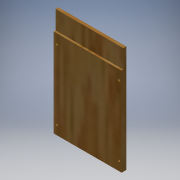
# Autodesk Inventor part: arduinoShelf
Saved by Autodesk Inventor 2016 (Build 200138000, 138)
## iProperties
Created: 2015-10-11
Part Number: arduinoShelf
Material: Plywood, Sheathing
Document SubType Name: Modeling
Designer: Artur
Density: 0.552 g/cm^3
Appearance: Plywood - New
Mass: 22.4443 g
Surface Area: 193.1 cm^2
Volume: 40.66 cm^3
Author: Artur
Autodesk Inventor part; units mm, degrees
ref_plane "YZ Plane" through (0, 0, 0) normal (1, 0, 0) x (0, 1, 0)
ref_plane "XZ Plane" through (0, 0, 0) normal (0, 1, 0) x (-1, 0, 0)
ref_plane "XY Plane" through (0, 0, 0) normal (0, 0, 1) x (1, 0, 0)
sketch "Sketch1" plane through (0, 0, 0) normal (0, 1, 0) x (-1, 0, 0)
  line L0 (0, 0) -> (-73, 0)
  line L1 (-73, 0) -> (-73, -115)
  line L2 (-73, -115) -> (0, -115)
  line L3 (0, -115) -> (0, 0)
  dimension "d0" = 115
  dimension "d1" = 73
  constraints: 8 end point, 2 parallel, 1 horizontal, 1 perpendicular
  measures "d0" distance of L2.end L0.start
  measures "d1" distance of L0.start L0.end
extrude "Extrusion1" add sketch "Sketch1" along normal blind 5
sketch "Sketch2" plane through (73, 0, 0) normal (1, 0, 0) x (0, 0, -1)
  line L0 (0, 0) -> (0, 5) construction
  line L1 (0, 0) -> (115, 0) construction
  line L2 (0, 2) -> (20, 2)
  line L3 (20, 2) -> (20, 0)
  line L4 (0, 2) -> (0, 0)
  line L5 (20, 0) -> (0, 0)
  dimension "d4" = 20
  dimension "d5" = 2
  constraints: 8 end point, 2 collinear, 2 perpendicular, 2 point on line
  measures "d4" distance of L2.start L2.end
  measures "d5" distance of L2.end L3.end
extrude "Extrusion2" cut sketch "Sketch2" against normal through all
sketch "Sketch3" plane through (0, 0, 0) normal (0, -1, 0) x (1, 0, 0)
  line L0 (0, -115) -> (0, 0) construction
  line L1 (73, -115) -> (0, -115) construction
  line L2 (0, 0) -> (73, 0) construction
  line L3 (73, 0) -> (73, -115) construction
  line L4 (73, -20) -> (0, -20) construction
  line L5 (36.5, -115) -> (36.5, -20) construction
  line L6 (73, -20) -> (0, -20) construction
  point P0 (3, -105)
  point P1 (3, -30)
  point P2 (70, -105)
  point P3 (70, -30)
  dimension "d8" = 10
  dimension "d9" = 3
  dimension "d10" = 3
  dimension "d11" = 10
  constraints: 2 end point, 2 midpoint, 2 symmetric about line
  measures "d8" distance from line of L1 point (3, -105)
  measures "d9" distance from line of point (3, -105) L0
  measures "d10" distance from line of L0 point (3, -30)
  measures "d11" distance from line of L4 point (3, -30)
hole "Hole1" at (3, 0, -105) at (3, 0, -30) at (70, 0, -105) at (70, 0, -30) direction (0, 1, 0) diameter 3 end through all
equation "\"d10\" = d9"
equation "\"d11\" = d8"
body "Solid1"
